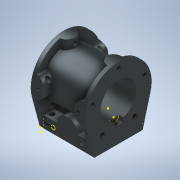
# Autodesk Inventor part: Part3
Saved by Autodesk Inventor 2020 (Build 240168000, 168)
## iProperties
Created: 2021-10-22
Part Number: Part3
Material: Iron, Cast
Document SubType Name: Modeling
Designer: simon.erikssonwestl
Density: 7.15 g/cm^3
Appearance: Iron Gray
Author: simon.erikssonwestl
Autodesk Inventor part; units mm, degrees
ref_plane "YZ Plane" through (0, 0, 0) normal (1, 0, 0) x (0, 1, 0)
ref_plane "XY Plane" through (0, 0, 0) normal (0, 0, 1) x (1, 0, 0)
ref_plane "UCS1: YZ Plane" through (0, 0, 0) normal (0.8660254, 0.5, 0) x (-0.5, 0.8660254, 0)
sketch "Sketch1" plane through (0, 0, 0) normal (1, 0, 0) x (0, 1, 0)
  circle A0 centre (20, 0) radius 17.5
  point P0 (0, 0)
  dimension "d0" = 35
  constraints: 1 centre point
  measures "d0" diameter of A0
sketch "Sketch2" plane through (0, 0, 0) normal (1, 0, 0) x (0, 1, 0)
  line L0 (0, 12.75) -> (0, -12.75)
  point P0 (0, 0)
  dimension "d1" = 25.5
  dimension "d2" = 12.75
  constraints: 2 end point, 1 vertical
  measures "d1" distance of L0.start L0.end
  measures "d2" distance of point (0, 0) L0.end
sketch "Sketch3" plane through (0, 0, 0) normal (1, 0, 0) x (0, 1, 0)
  circle A0 centre (20, 0) radius 17.5 projected
  line L0 (0, 12.75) -> (0, -12.75) projected
  line L1 (0, -12.75) -> (15.4622, -16.9014)
  line L2 (0, 12.75) -> (15.4622, 16.9014)
  point P0 (0, 0)
  constraints: 4 end point, 2 point on circle, 2 tangent
extrude "Extrusion1" add sketch "Sketch3" along normal blind 2
sketch "Sketch4" plane through (2, 0, 0) normal (1, 0, 0) x (0, 0, -1)
  arc A0 (16.9014, 15.4622) -> (-16.9014, 15.4622) centre (0, 20) ccw projected
  circle A1 centre (0, 20) radius 12.75
  line L0 (-6.75, 6) -> (6.75, 6)
  line L1 (-12.75, 0) -> (12.75, 0) projected
  line L2 (-6.75, 6) -> (-6.75, 9.1833)
  line L3 (6.75, 6) -> (6.75, 9.1833)
  line L4 (-12.75, 6) -> (12.75, 6)
  line L5 (12.75, 6) -> (12.75, 0)
  line L6 (12.75, 0) -> (-12.75, 0)
  line L7 (-12.75, 0) -> (-12.75, 6)
  line L8 (-6.75, 9.1833) -> (6.75, 9.1833)
  point P0 (0, 0)
  dimension "d5" = 25.5
  dimension "d6" = 13.5
  dimension "d7" = 6.75
  dimension "d8" = 6
  dimension "d9" = 25.5
  dimension "d10" = 6
  dimension "d11" = 0
  dimension "d12" = 90
  constraints: 16 end point, 2 horizontal, 2 parallel, 2 point on circle, 1 centre point, 1 coincident, 1 perpendicular, 1 vertical
  measures "d5" diameter of A1
  measures "d6" distance of L0.start L0.end
  measures "d7" horizontal distance of point (0, 0) L0.start
  measures "d8" distance between parallel lines of L1 L0
  measures "d9" distance of L5.end L6.end
  measures "d10" distance of L4.end L5.end
  measures "d11" distance of L1.start L6.end
  measures "d12" angle of L4 L3
extrude "Extrusion2" add sketch "Sketch4" along normal blind 25
sketch "Sketch5" plane through (27, 0, 0) normal (1, 0, 0) x (0, 0, -1)
  arc A0 (16.9014, 15.4622) -> (-16.9014, 15.4622) centre (0, 20) ccw projected
  line L0 (-16.9014, 15.4622) -> (-12.75, 0) projected
  line L1 (12.75, 0) -> (16.9014, 15.4622) projected
  circle A1 centre (0, 20) radius 17.5
  line L2 (-12.75, 0) -> (12.75, 0) projected
  line L3 (-12.75, 0) -> (-16.9014, 15.4622)
  line L4 (12.75, 0) -> (16.9014, 15.4622)
  point P0 (0, 0)
  dimension "d15" = 35
  constraints: 4 end point, 2 point on circle, 2 tangent, 1 centre point, 1 coincident
  measures "d15" diameter of A1
extrude "Extrusion3" add sketch "Sketch5" along normal blind 2
sketch "Sketch6" plane through (2, 0, -12.75) normal (0, 0, -1) x (-1, 0, 0)
  arc A0 (-7, 6) -> (-18, 6) centre (-12.5, 6) ccw
  line L0 (0, 6) -> (-25, 6) projected
  point P0 (2, 0)
  dimension "d18" = 5.5
  constraints: 2 point on circle, 1 centre point
  measures "d18" radius of A0
extrude "Extrusion4" add sketch "Sketch6" against normal blind 25.5
sketch "Sketch7" plane through (0, 0, -12.75) normal (0, -1, 0) x (1, 0, 0)
  line L0 (11, 16.25) -> (9, 16.25)
  line L1 (9, 16.25) -> (9, 9.25)
  line L2 (9, 9.25) -> (11, 9.25)
  line L3 (11, 9.25) -> (11, 16.25)
  line L4 (0, 25.5) -> (0, 0) projected
  line L5 (2, 0) -> (27, 0) projected
  line L6 (2, 25.5) -> (27, 25.5) projected
  line L7 (13, 16.25) -> (16, 16.25)
  line L8 (16, 16.25) -> (16, 9.25)
  line L9 (16, 9.25) -> (13, 9.25)
  line L10 (13, 9.25) -> (13, 16.25)
  line L11 (20, 16.25) -> (18, 16.25)
  line L12 (18, 16.25) -> (18, 9.25)
  line L13 (18, 9.25) -> (20, 9.25)
  line L14 (20, 9.25) -> (20, 16.25)
  point P0 (0, 12.75)
  dimension "d21" = 2
  dimension "d22" = 7
  dimension "d23" = 9
  dimension "d24" = 9.25
  dimension "d25" = 9.25
  dimension "d26" = 3
  dimension "d27" = 2
  dimension "d28" = 9.25
  dimension "d29" = 9.25
  dimension "d30" = 2
  dimension "d31" = 20
  dimension "d32" = 9.25
  dimension "d33" = 9.25
  constraints: 24 end point, 6 parallel, 3 horizontal, 3 perpendicular
  measures "d21" distance of L2.end L1.end
  measures "d22" distance of L1.end L0.end
  measures "d23" distance between parallel lines of L4 L1
  measures "d24" distance between parallel lines of L5 L2
  measures "d25" distance between parallel lines of L6 L0
  measures "d26" distance of L8.end L9.end
  measures "d27" distance between parallel lines of L10 L3
  measures "d28" distance between parallel lines of L6 L7
  measures "d29" distance between parallel lines of L5 L9
  measures "d30" distance between parallel lines of L8 L12
  measures "d31" distance between parallel lines of L4 L14
  measures "d32" distance between parallel lines of L6 L11
  measures "d33" distance between parallel lines of L5 L13
extrude "Extrusion5" cut sketch "Sketch7" against normal blind 5
sketch "Sketch8" plane through (2, 0, 0) normal (1, 0, 0) x (0, 0, -1)
  arc A0 (16.9014, 15.4622) -> (-16.9014, 15.4622) centre (0, 20) ccw projected
  arc A1 (16.9014, 15.4622) -> (-16.9014, 15.4622) centre (0, 20) ccw projected
  arc A2 (6.75, 9.1833) -> (-6.75, 9.1833) centre (0, 20) ccw projected
  line L0 (-4, 37.0367) -> (-4, 32.1063)
  line L1 (4, 37.0367) -> (4, 32.1063)
  point P0 (0, 0)
  dimension "d36" = 4
  dimension "d37" = 8
  constraints: 4 end point, 4 point on circle, 1 vertical
  measures "d36" horizontal distance of point (0, 0) L0.start
  measures "d37" distance of L0.start L1.start
extrude "Extrusion6" add sketch "Sketch8" along normal blind 4
fillet "Fillet1" radius 4 2 edges at (6, 34.5715, 4) (6, 34.5715, -4)
sketch "Sketch9" plane through (27, 0, 0) normal (-1, 0, 0) x (0, 0, 1)
  arc A0 (16.9014, 15.4622) -> (-16.9014, 15.4622) centre (0, 20) ccw projected
  line L0 (-4, 37.0367) -> (-4, 32.1063)
  arc A1 (6.75, 9.1833) -> (-6.75, 9.1833) centre (0, 20) ccw projected
  line L1 (4, 37.0367) -> (4, 32.1063)
  point P0 (0, 0)
  dimension "d41" = 4
  dimension "d42" = 8
  constraints: 4 end point, 4 point on circle, 1 parallel, 1 vertical
  measures "d41" horizontal distance of point (0, 0) L0.start
  measures "d42" distance of L1.start L0.start
extrude "Extrusion7" add sketch "Sketch9" along normal blind 4
fillet "Fillet2" radius 4 2 edges at (23, 34.5715, -4) (23, 34.5715, 4)
sketch "Sketch10" plane through (0, 0, -12.75) normal (0, -1, 0) x (1, 0, 0)
  line L0 (2, 0) -> (27, 0) projected
  line L1 (29, 25.5) -> (29, 0) projected
  line L2 (2, 25.5) -> (27, 25.5) projected
  line L3 (0, 25.5) -> (0, 0) projected
  point P0 (0, 12.75)
  point P1 (25.25, 2.75)
  point P2 (3.75, 2.75)
  point P3 (3.75, 22.75)
  point P4 (25.25, 22.75)
  dimension "d46" = 2.75
  dimension "d47" = 3.75
  dimension "d48" = 20
  dimension "d49" = 21.5
  dimension "d50" = 20
  dimension "d51" = 3.75
  dimension "d52" = 2.75
  dimension "d53" = 3.75
  measures "d46" distance from line of point (25.25, 2.75) L0
  measures "d47" distance from line of L1 point (25.25, 2.75)
  measures "d48" distance of point (25.25, 22.75) point (25.25, 2.75)
  measures "d49" distance of point (3.75, 22.75) point (25.25, 22.75)
  measures "d50" distance of point (3.75, 2.75) point (3.75, 22.75)
  measures "d51" distance from line of L1 point (25.25, 22.75)
  measures "d52" distance from line of L2 point (3.75, 22.75)
  measures "d53" distance from line of L3 point (3.75, 2.75)
hole "Hole1" at (25.25, 0, -10) at (3.75, 0, -10) at (3.75, 0, 10) at (25.25, 0, 10) direction (0, 1, 0) diameter 2.5 depth 7 tip angle 118
thread "Thread1" size "M2.5x0.45" class "6H" standard "ANSI Metric M Profile" full length
thread "Thread2" size "M2.5x0.45" class "6H" standard "ANSI Metric M Profile" full length
thread "Thread3" size "M2.5x0.45" class "6H" standard "ANSI Metric M Profile" full length
thread "Thread4" size "M2.5x0.45" class "6H" standard "ANSI Metric M Profile" full length
sketch "Sketch11" plane through (0, 0, 0) normal (-1, 0, 0) x (0, 0, 1)
  arc A0 (16.9014, 15.4622) -> (-16.9014, 15.4622) centre (0, 20) ccw projected
  circle A1 centre (0, 20) radius 9.5
  point P0 (0, 0)
  dimension "d69" = 19
  constraints: 1 centre point, 1 coincident
  measures "d69" diameter of A1
extrude "Extrusion8" cut sketch "Sketch11" against normal through all
sketch "Sketch12" plane through (0, 0, 0) normal (-1, 0, 0) x (0, 0, 1)
  circle A0 centre (0, 20) radius 9.5 projected
  circle A1 centre (0, 20) radius 9.5 projected
  arc A2 (-2.5, 10.8348) -> (2.5, 10.8348) centre (0, 10.8348) ccw
  point P0 (0, 0)
  dimension "d72" = 2.5
  dimension "d73" = 5
  dimension "d74" = 2.5
  constraints: 4 point on circle, 1 centre point
  measures "d72" horizontal distance of A0.centre A1.start
  measures "d73" distance of A1.end A1.start
  measures "d74" radius of A2
extrude "Extrusion9" cut sketch "Sketch12" against normal blind 2.5 contours A0 A2
sketch "Sketch13" plane through (29, 0, 0) normal (1, 0, 0) x (0, 0, -1)
  circle A0 centre (0, 20) radius 9.5 projected
  arc A1 (-2.5, 10.8348) -> (2.5, 10.8348) centre (0, 10.8348) ccw projected
  arc A2 (-2.5, 10.8348) -> (2.5, 10.8348) centre (0, 10.8348) ccw
  point P0 (0, 0)
  dimension "d77" = 2.5
  dimension "d78" = 5
  constraints: 5 point on circle, 1 centre point, 1 concentric
  measures "d77" horizontal distance of A0.centre A0.start
  measures "d78" distance of A0.end A0.start
extrude "Extrusion10" cut sketch "Sketch13" against normal blind 2.5 contours A0 A1
sketch "Sketch14" plane through (2.5, 0, 0) normal (-1, 0, 0) x (0, 0, 1)
  point P0 (0, 0)
sketch "Sketch15" plane through (2.5, 0, 0) normal (-1, 0, 0) x (0, 0, 1)
  arc A0 (-2.5, 10.8348) -> (2.5, 10.8348) centre (0, 10.8348) ccw projected
  line L0 (0, 8.3348) -> (-0.2827, 8.3348)
  point P0 (0, 0)
  constraints: 2 end point, 1 horizontal, 1 point on circle, 1 tangent
ref_plane "Work Plane1" through (2.5, 8.3348, 0) normal (0.8660254, -0.5, 0) x (0, 0, -1)
sketch "Sketch16" plane through (2.5, 8.3348, 0) normal (0.8660254, -0.5, 0) x (0, 0, -1)
  circle A0 centre (0, 0) radius 1
  point P0 (0, -8.4682)
  dimension "d82" = 2
  constraints: 2 coincident, 1 centre point
  measures "d82" diameter of A0
extrude "Extrusion11" cut sketch "Sketch16" along normal blind 9 and the other way blind 4
sketch "Sketch19" plane through (26.5, 0, 0) normal (1, 0, 0) x (0, 0, -1)
  arc A0 (-2.5, 10.8348) -> (2.5, 10.8348) centre (0, 10.8348) ccw projected
  line L0 (0, 8.3348) -> (-0.5888, 8.3348)
  point P0 (0, 0)
  constraints: 2 end point, 1 horizontal, 1 point on circle, 1 tangent
ref_plane "Work Plane2" through (26.5, 8.3348, 0) normal (-0.8660254, -0.5, 0) x (0, 0, 1)
sketch "Sketch20" plane through (26.5, 8.3348, 0) normal (-0.8660254, -0.5, 0) x (0, 0, 1)
  point P0 (0, 6.0318)
sketch "Sketch23" plane through (2, 0, -12.75) normal (0, 0, -1) x (-1, 0, 0)
  arc A0 (-7, 6) -> (-18, 6) centre (-12.5, 6) ccw projected
  point P0 (2, 0)
hole "Hole3" at (14.5, 6, -12.75) direction (0, 0, 1) diameter 3 depth 16 tip angle 118 counterbore diameter 5 counterbore depth 5
sketch "Sketch24" plane through (29, 15.4622, -16.9014) normal (0, -0.2593055, -0.9657954) x (-1, 0, 0)
  line L0 (0, -13.0098) -> (2, -13.0098)
  line L1 (2, -16.0098) -> (0, -16.0098) projected
  point P0 (29, -19.3159)
  dimension "d115" = 3
  constraints: 2 end point
  measures "d115" distance between parallel lines of L0 L1
sketch "Sketch25" plane through (2, 0, -12.75) normal (0, 0, -1) x (-1, 0, 0)
  line L0 (-27, 2.8974) -> (-25, 2.8974) projected
  line L1 (-25, 2.8974) -> (-21.7388, 2.8974)
  point P0 (2, 0)
  constraints: 2 end point, 1 horizontal
ref_plane "Work Plane3" through (27, 2.8974, -12.75) normal (0, 0.2593055, 0.9657954) x (-1, 0, 0)
sketch "Sketch26" plane through (27, 2.8974, -12.75) normal (0, 0.2593055, 0.9657954) x (-1, 0, 0)
  line L0 (0, 2.7983) -> (0, -13.2115) projected
  line L1 (-2, 2.7983) -> (-2, -13.2115) projected
  line L2 (27, 2.7983) -> (27, -13.2115) projected
  point P0 (27, 6.1044)
  point P1 (5, 0)
  point P2 (20, 0)
  dimension "d118" = 7
  dimension "d119" = 7
  measures "d118" distance from line of L1 point (5, 0)
  measures "d119" distance from line of L2 point (20, 0)
hole "Hole4" at (22, 2.8974, -12.75) at (7, 2.8974, -12.75) direction (0, 0.2593055, 0.9657954) diameter 2 depth 7 tip angle 118
sketch "Sketch27" plane through (27, 2.8974, -12.75) normal (0, 0.2593055, 0.9657954) x (-1, 0, 0)
  arc A0 (6, 0) -> (4, 0) centre (5, 0) ccw projected
  arc A1 (4, 0) -> (6, 0) centre (5, 0) ccw projected
  arc A2 (19, 0) -> (21, 0) centre (20, 0) ccw projected
  arc A3 (21, 0) -> (19, 0) centre (20, 0) ccw projected
  point P0 (27, 6.1044)
extrude "Extrusion14" cut sketch "Sketch27" against normal blind 1
sketch "Sketch28" plane through (0, 15.4622, 16.9014) normal (0, -0.2593055, 0.9657954) x (1, 0, 0)
  line L0 (0, -16.0098) -> (2, -16.0098) projected
  point P0 (0, -19.3159)
  point P1 (2, -13.0098)
  dimension "d129" = 3
  measures "d129" distance from line of L0 point (2, -13.01)
sketch "Sketch29" plane through (2, 0, 12.75) normal (0, 0, 1) x (1, 0, 0)
  ellipse E0 centre (5, 2.8974) end of major axis (5, 1.862) minor radius 1 projected
  line L0 (0, 2.8974) -> (5, 2.8974)
  point P0 (-2, 0)
  constraints: 2 end point, 1 other
ref_plane "Work Plane4" through (2, 2.8974, 12.75) normal (0, 0.2593055, -0.9657954) x (1, 0, 0)
sketch "Sketch30" plane through (2, 2.8974, 12.75) normal (0, 0.2593055, -0.9657954) x (1, 0, 0)
  line L0 (0, 0) -> (5, 0) projected
  line L1 (-2, -13.2115) -> (-2, 2.7983) projected
  line L2 (27, -13.2115) -> (27, 2.7983) projected
  point P0 (-2, 6.1044)
  point P1 (5, 0)
  point P2 (20, 0)
  dimension "d131" = 7
  dimension "d132" = 7
  measures "d131" distance from line of L1 point (5, 0)
  measures "d132" distance from line of L2 point (20, 0)
hole "Hole5" at (22, 2.8974, 12.75) at (7, 2.8974, 12.75) direction (0, 0.2593055, -0.9657954) diameter 2 depth 7 tip angle 118
sketch "Sketch31" plane through (2, 2.8974, 12.75) normal (0, 0.2593055, -0.9657954) x (1, 0, 0)
  arc A0 (4, 0) -> (6, 0) centre (5, 0) ccw projected
  circle A1 centre (5, 0) radius 1 projected
  arc A2 (19, 0) -> (21, 0) centre (20, 0) ccw projected
  arc A3 (21, 0) -> (19, 0) centre (20, 0) ccw projected
  point P0 (-2, 6.1044)
extrude "Extrusion15" cut sketch "Sketch31" against normal blind 1
sketch "Sketch32" plane through (26.5, 8.3348, 0) normal (-0.8660254, -0.5, 0) x (0, 0, 1)
  ellipse E0 centre (0, 2.1651) end of major axis (2.5, 2.1651) minor radius 2.1651 (-2.5, 2.1651) -> (2.5, 2.1651) ccw projected
  circle A0 centre (0, 0) radius 1
  point P0 (0, 6.0318)
  dimension "d142" = 2
  constraints: 1 centre point, 2 other
  measures "d142" diameter of A0
extrude "Extrusion16" cut sketch "Sketch32" along normal blind 9 and the other way blind 4
sketch "Sketch33" plane through (29, 0, 0) normal (1, 0, 0) x (0, 0, -1)
  circle A0 centre (0, 34.5) radius 1.25
  arc A1 (2.5, 10.8348) -> (-2.5, 10.8348) centre (0, 20) ccw projected
  circle A2 centre (-13.7903, 24.4807) radius 1.25
  circle A3 centre (-8.5229, 8.2693) radius 1.25
  circle A4 centre (8.5229, 8.2693) radius 1.25
  circle A5 centre (13.7903, 24.4807) radius 1.25
  point P0 (0, 0)
  dimension "d147" = 2.5
  dimension "d148" = 14.5
  dimension "d151" = 360
  constraints: 5 centre point, 11 other
  measures "d147" diameter of A0
  measures "d148" distance of A1.centre A0.centre
extrude "Extrusion17" cut sketch "Sketch33" against normal blind 6
sketch "Sketch34" plane through (0, 0, 0) normal (-1, 0, 0) x (0, 0, 1)
  circle A0 centre (0, 34.5) radius 1.25 projected
  circle A1 centre (0, 34.5) radius 1.25
  arc A2 (2.5, 10.8348) -> (-2.5, 10.8348) centre (0, 20) ccw projected
  circle A3 centre (-13.7903, 24.4807) radius 1.25
  circle A4 centre (-8.5229, 8.2693) radius 1.25
  circle A5 centre (8.5229, 8.2693) radius 1.25
  circle A6 centre (13.7903, 24.4807) radius 1.25
  point P0 (0, 0)
  dimension "d157" = 360
  constraints: 5 centre point, 3 coincident, 14 other
extrude "Extrusion18" cut sketch "Sketch34" against normal blind 6
thread "Thread5" size "M2.5x0.45" class "6H" standard "ANSI Metric M Profile" full length
thread "Thread6" size "M2.5x0.45" class "6H" standard "ANSI Metric M Profile" full length
thread "Thread7" size "M2.5x0.45" class "6H" standard "ANSI Metric M Profile" full length
thread "Thread8" size "M2.5x0.45" class "6H" standard "ANSI Metric M Profile" full length
thread "Thread9" size "M2.5x0.45" class "6H" standard "ANSI Metric M Profile" full length
thread "Thread10" size "M2.5x0.45" class "6H" standard "ANSI Metric M Profile" full length
thread "Thread11" size "M2.5x0.45" class "6H" standard "ANSI Metric M Profile" full length
thread "Thread12" size "M2.5x0.45" class "6H" standard "ANSI Metric M Profile" full length
thread "Thread13" size "M2.5x0.45" class "6H" standard "ANSI Metric M Profile" full length
thread "Thread14" size "M2.5x0.45" class "6H" standard "ANSI Metric M Profile" full length
sketch "Sketch35" plane through (2, 0, 0) normal (1, 0, 0) x (0, 0, -1)
  arc A0 (16.9014, 15.4622) -> (-16.9014, 15.4622) centre (0, 20) ccw projected
  arc A1 (2.5, 10.8348) -> (-2.5, 10.8348) centre (0, 20) ccw projected
  line L0 (-16.9014, 15.4622) -> (-12.75, 0) projected
  line L1 (-16.9014, 15.4622) -> (-8.3461, 15.4622)
  line L2 (-16.2632, 26.4622) -> (-6.9635, 26.4622)
  line L3 (12.75, 0) -> (16.9014, 15.4622) projected
  line L4 (16.2632, 26.4622) -> (6.9635, 26.4622)
  line L5 (16.9014, 15.4622) -> (8.3461, 15.4622)
  point P0 (0, 0)
  point P1 (16.9014, 15.4622)
  point P2 (-16.9014, 15.4622)
  dimension "d181" = 11
  dimension "d182" = 11
  constraints: 8 end point, 6 point on circle, 2 coincident, 2 horizontal, 2 parallel
  measures "d181" vertical distance of L0.start L2.start
  measures "d182" vertical distance of L5.start L4.start
extrude "Extrusion19" add sketch "Sketch35" along normal blind 4 contours L5 A1 L4 A0 | L2 A1 L1 A0
sketch "Sketch36" plane through (27, 0, 0) normal (-1, 0, 0) x (0, 0, 1)
  line L0 (-12.75, 0) -> (-16.9014, 15.4622) projected
  arc A0 (16.9014, 15.4622) -> (-16.9014, 15.4622) centre (0, 20) ccw projected
  line L1 (-16.2632, 26.4622) -> (-6.9635, 26.4622)
  arc A1 (2.5, 10.8348) -> (-2.5, 10.8348) centre (0, 20) ccw projected
  line L2 (-16.9014, 15.4622) -> (-8.342, 15.4622)
  line L3 (16.2704, 26.444) -> (7.3655, 26)
  line L4 (16.9014, 15.4622) -> (12.75, 0) projected
  line L5 (16.9014, 15.4622) -> (8.3461, 15.4622)
  point P0 (0, 0)
  point P1 (16.9014, 15.4622)
  point P2 (-8.3461, 15.4622)
  dimension "d186" = 11
  dimension "d187" = 11
  constraints: 8 end point, 5 point on circle, 3 horizontal, 1 coincident
  measures "d186" distance of point (16.901, 15.462) L3.start
  measures "d187" vertical distance of L1.start L0.end
extrude "Extrusion20" add sketch "Sketch36" along normal blind 4 contours L5 A1 L3 A0 | L1 A1 L2 A0
fillet "Fillet4" radius 4 4 edges at (23, 26.3163, 13.7089) (23, 15.4622, 14.4083) (23, 15.4622, -14.4083) (23, 26.4622, -13.6271)
sketch "Sketch37" plane through (27, 24.4807, 13.7903) normal (1, 0, 0) x (0, 0, -1)
  circle A0 centre (0, 0) radius 1.25 projected
  circle A1 centre (27.5806, 0) radius 1.25 projected
  point P0 (13.7903, -24.4807)
extrude "Extrusion21" cut sketch "Sketch37" against normal blind 4
sketch "Sketch38" plane through (2, 24.4807, 13.7903) normal (-1, 0, 0) x (0, 0, 1)
  circle A0 centre (0, 0) radius 1.25 projected
  circle A1 centre (-27.5806, 0) radius 1.25 projected
  point P0 (-13.7903, -24.4807)
extrude "Extrusion22" cut sketch "Sketch38" against normal blind 4
fillet "Fillet5" radius 4 4 edges at (6, 26.4622, 13.6271) (6, 15.4622, 14.4083) (6, 26.4622, -13.6271) (6, 15.4622, -14.4083)
sketch "Sketch39" plane through (6, 0, 0) normal (1, 0, 0) x (0, 0, -1)
  arc A0 (17.4917, 19.4622) -> (17.3259, 22.4622) centre (0, 20) ccw projected
  line L0 (12.51, 22.4622) -> (17.3259, 22.4622) projected
  line L1 (17.4917, 19.4622) -> (12.7387, 19.4622) projected
  point P0 (0, 0)
  point P1 (17.4735, 20.9622)
  dimension "d196" = 1.5
  dimension "d197" = 1.5
  constraints: 1 point on circle
  measures "d196" distance from line of L0 point (17.474, 20.962)
  measures "d197" distance from line of L1 point (17.474, 20.962)
ref_plane "Work Plane5" through (6, 20.9622, -17.4735) normal (0, 0.0549803, -0.9984874) x (-1, 0, 0)
sketch "Sketch40" plane through (6, 20.9622, -17.4735) normal (0, 0.0549803, -0.9984874) x (-1, 0, 0)
  line L0 (6, -5.4602) -> (4, -5.4602) projected
  line L1 (6, 17.5) -> (6, -3.6017) projected
  line L2 (6, -3.6017) -> (4, -3.6017) projected
  line L3 (0, 3.411) -> (0, 0.4247) projected
  line L4 (4, 17.2309) -> (4, 7.3465) projected
  line L5 (4, 5.5582) -> (4, 16.791) projected
  line L6 (0, -1.4987) -> (0, 1.5058) projected
  line L7 (6, 17.5) -> (6, 17.5) projected
  line L8 (-21, 5.5582) -> (-21, 16.791) projected
  line L9 (-21, 17.2309) -> (-21, 7.3288) projected
  line L10 (-17, 0.4247) -> (-17, 3.4401) projected
  line L11 (-21, -3.6017) -> (-23, -3.6017) projected
  line L12 (-23, -5.4602) -> (-23, -3.6017) projected
  line L13 (-21, -5.4602) -> (-23, -5.4602) projected
  line L14 (-17, 1.5058) -> (-17, -1.4987) projected
  line L15 (-23, 17.5) -> (-23, -5.4602) projected
  point P0 (6, -19.9697)
  point P1 (2, 0.0398)
  point P2 (-19, 0.0398)
  dimension "d198" = 4
  dimension "d199" = 5.5
  dimension "d200" = 5.5
  dimension "d201" = 4
  constraints: 12 other
  measures "d198" distance from line of L7 point (2, 0.04)
  measures "d199" distance from line of point (2, 0.04) L0
  measures "d200" distance from line of L13 point (-19, 0.04)
  measures "d201" distance from line of L15 point (-19, 0.04)
hole "Hole6" at (4, 21.0019, -17.4713) at (25, 21.0019, -17.4713) direction (0, -0.0549803, 0.9984874) diameter 2 depth 5 tip angle 118
sketch "Sketch41" plane through (6, 0, 0) normal (1, 0, 0) x (0, 0, -1)
  arc A0 (-17.3259, 22.4622) -> (-17.4917, 19.4622) centre (0, 20) ccw projected
  line L0 (-17.3259, 22.4622) -> (-12.51, 22.4622) projected
  point P0 (0, 0)
  point P1 (-17.4735, 20.9622)
  dimension "d209" = 1.5
  constraints: 1 point on circle
  measures "d209" distance from line of L0 point (-17.474, 20.962)
ref_plane "Work Plane6" through (6, 20.9622, 17.4735) normal (0, 0.0549803, 0.9984874) x (-1, 0, 0)
sketch "Sketch42" plane through (6, 20.9622, 17.4735) normal (0, 0.0549803, 0.9984874) x (-1, 0, 0)
  line L0 (0, 1.4987) -> (0, -1.5058) projected
  line L1 (-17, -1.5354) -> (-17, 1.4987) projected
  point P0 (6, 19.9697)
  point P1 (2, -0.0058)
  point P2 (-19, -0.0013)
  dimension "d210" = 2
  dimension "d211" = 1.5
  dimension "d212" = 2
  dimension "d213" = 1.5
  measures "d210" distance from line of L0 point (2, -0.006)
  measures "d211" vertical distance of point (2, -0.006) L0.end
  measures "d212" distance from line of L1 point (-19, -0.001)
  measures "d213" vertical distance of L1.end point (-19, -0.001)
hole "Hole7" at (4, 20.968, 17.4732) at (25, 20.9634, 17.4735) direction (0, -0.0549803, -0.9984874) diameter 2 depth 5 tip angle 118
body "Solid1"
